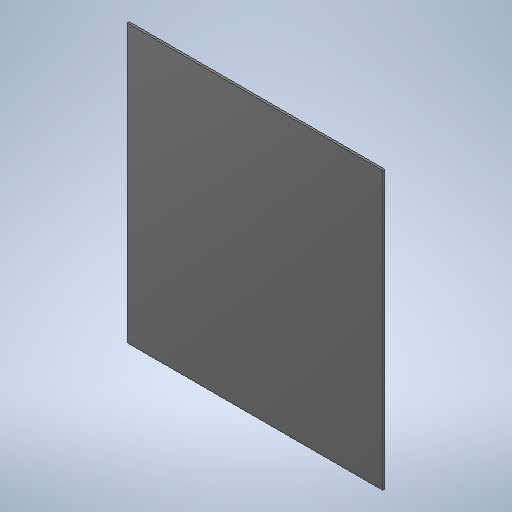
# Autodesk Inventor part: Foam Sheet Side
Saved by Autodesk Inventor 2026.2 (Build 302298010, 298A)
## iProperties
Created: 2026-06-07
Part Number: Foam Sheet Side
Material: PVC-Piping
Document SubType Name: Modeling
Designer: chanh
Density: 1.4 g/cm^3
Appearance: Smooth - White
Author: chanh
Autodesk Inventor part; units mm, degrees
ref_plane "YZ Plane" through (0, 0, 0) normal (1, 0, 0) x (0, 1, 0)
ref_plane "XZ Plane" through (0, 0, 0) normal (0, 1, 0) x (-1, 0, 0)
ref_plane "XY Plane" through (0, 0, 0) normal (0, 0, 1) x (1, 0, 0)
sketch "Sketch1" plane through (0, 0, 0) normal (0, 0, 1) x (1, 0, 0)
  line L0 (-300, -325) -> (300, -325)
  line L1 (300, -325) -> (300, 325)
  line L2 (300, 325) -> (-300, 325)
  line L3 (-300, 325) -> (-300, -325)
  line L4 (-300, -325) -> (300, 325) construction
  line L5 (300, -325) -> (-300, 325) construction
  point P0 (0, 0)
  dimension "d0" = 600
  dimension "d1" = 650
  constraints: 12 end point, 2 midpoint, 2 parallel, 1 horizontal, 1 perpendicular
  measures "d0" distance of L1.end L2.end
  measures "d1" distance of L0.end L1.end
extrude "Extrusion1" add sketch "Sketch1" along normal blind 5
body "Solid1"
